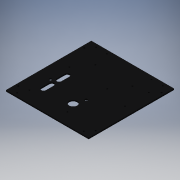
# Autodesk Inventor part: SwarmieTopPlate
Saved by Autodesk Inventor 2016 (Build 200138000, 138)
## iProperties
Created: 2015-05-25
Part Number: SwarmieTopPlate
Material: Generic
Document SubType Name: Modeling
Designer: Karl
Density: 1 g/cm^3
Appearance: Glossy - Black
Author: Karl
Autodesk Inventor part; units mm, degrees
ref_plane "YZ Plane" through (0, 0, 0) normal (1, 0, 0) x (0, 1, 0)
ref_plane "XZ Plane" through (0, 0, 0) normal (0, 1, 0) x (-1, 0, 0)
ref_plane "XY Plane" through (0, 0, 0) normal (0, 0, 1) x (1, 0, 0)
sketch "Sketch1" plane through (0, 0, 0) normal (0, 1, 0) x (-1, 0, 0)
  line L0 (98.0186, -101.2063) -> (-98.0186, -101.2063)
  line L1 (-98.0186, -101.2063) -> (-98.0186, 101.2063)
  line L2 (-98.0186, 101.2063) -> (98.0186, 101.2063)
  line L3 (98.0186, 101.2063) -> (98.0186, -101.2063)
  line L4 (98.0186, -101.2063) -> (-98.0186, 101.2063) construction
  line L5 (-98.0186, -101.2063) -> (98.0186, 101.2063) construction
  point P0 (0, 0)
  dimension "d0" = 196.0372
  dimension "d1" = 202.4126
  constraints: 12 end point, 2 midpoint, 2 parallel, 1 horizontal, 1 perpendicular
  measures "d0" distance of L1.end L2.end
  measures "d1" distance of L0.end L1.end
extrude "Extrusion1" add sketch "Sketch1" along normal blind 3
sketch "Sketch2" plane through (0, 3, 0) normal (0, 1, 0) x (1, 0, 0)
  line L0 (98.0186, 101.2063) -> (-98.0186, 101.2063) projected
  line L1 (-98.0186, 101.2063) -> (-98.0186, -101.2063) projected
  line L2 (-98.0186, -101.2063) -> (98.0186, -101.2063) projected
  line L3 (98.0186, -101.2063) -> (98.0186, 101.2063) projected
  point P0 (0, 0)
  point P1 (-91.6686, 78.0923)
  point P2 (91.6686, 78.0923)
  point P3 (-91.6686, -78.0923)
  point P4 (91.6686, -78.0923)
  dimension "d4" = 23.114
  dimension "d5" = 23.114
  dimension "d6" = 6.35
  dimension "d7" = 6.35
  constraints: 2 horizontal alignment, 2 vertical alignment
  measures "d4" distance from line of L0 point (-91.669, 78.092)
  measures "d5" distance from line of L2 point (-91.669, -78.092)
  measures "d6" distance from line of L1 point (-91.669, 78.092)
  measures "d7" distance from line of L3 point (91.669, 78.092)
hole "Hole1" at (-91.6686, 3, -78.0923) at (91.6686, 3, -78.0923) at (-91.6686, 3, 78.0923) at (91.6686, 3, 78.0923) direction (0, -1, 0) diameter 3.81 end through all
sketch "Sketch5" plane through (0, 3, 0) normal (0, 1, 0) x (1, 0, 0)
  line L0 (-98.0186, 101.2063) -> (-98.0186, -101.2063) projected
  line L1 (-98.0186, -101.2063) -> (98.0186, -101.2063) projected
  point P0 (0, 0)
  point P1 (-70.0786, -73.2663)
  point P2 (19.8374, -73.2663)
  point P3 (19.8374, 21.2217)
  point P4 (-70.0786, 21.2217)
  dimension "d44" = 27.94
  dimension "d45" = 27.94
  dimension "d46" = 89.916
  dimension "d47" = 94.488
  constraints: 2 horizontal alignment, 2 vertical alignment
  measures "d44" distance from line of L1 point (-70.079, -73.266)
  measures "d45" distance from line of L0 point (-70.079, -73.266)
  measures "d46" distance of point (19.837, -73.266) point (-70.079, -73.266)
  measures "d47" distance of point (-70.079, 21.222) point (-70.079, -73.266)
hole "Hole4" at (-70.0786, 3, 73.2663) at (19.8374, 3, 73.2663) at (19.8374, 3, -21.2217) at (-70.0786, 3, -21.2217) direction (0, -1, 0) diameter 3.302 end through all
sketch "Sketch6" plane through (0, 3, 0) normal (0, 1, 0) x (1, 0, 0)
  circle A0 centre (-70.0786, -73.2663) radius 1.651 projected
  circle A1 centre (19.8374, -73.2663) radius 1.651 projected
  point P0 (0, 0)
  point P1 (-67.2846, -26.0223)
  point P2 (17.0434, -26.0223)
  dimension "d55" = 2.794
  dimension "d56" = 2.794
  dimension "d57" = 47.244
  constraints: 1 horizontal alignment
  measures "d55" horizontal distance of point (-67.285, -26.022) A0.centre
  measures "d56" horizontal distance of A1.centre point (17.043, -26.022)
  measures "d57" vertical distance of point (-67.285, -26.022) A0.centre
hole "Hole5" at (-67.2846, 3, 26.0223) at (17.0434, 3, 26.0223) direction (0, -1, 0) diameter 6.35 end through all
sketch "Sketch10" plane through (0, 3, 0) normal (0, 1, 0) x (1, 0, 0)
  line L0 (98.0186, 101.2063) -> (-98.0186, 101.2063) projected
  line L1 (98.0186, -101.2063) -> (98.0186, 101.2063) projected
  line L2 (0, 56.7563) -> (0, 92.8243)
  point P0 (0, 0)
  point P1 (-52.8574, 92.8243)
  point P2 (-43.9674, 56.7563)
  point P3 (52.8574, 92.8243)
  point P4 (43.9674, 56.7563)
  dimension "d91" = 52.8574
  dimension "d92" = 8.382
  dimension "d93" = 36.068
  dimension "d94" = 8.89
  constraints: 2 end point, 2 symmetric about line, 1 parallel
  measures "d91" horizontal distance of point (-52.857, 92.824) point (0, 0)
  measures "d92" distance from line of L0 point (-52.857, 92.824)
  measures "d93" vertical distance of point (-43.967, 56.756) point (-52.857, 92.824)
  measures "d94" horizontal distance of point (-43.967, 56.756) point (-52.857, 92.824)
hole "Hole8" at (-52.8574, 3, -92.8243) at (-43.9674, 3, -56.7563) at (52.8574, 3, -92.8243) at (43.9674, 3, -56.7563) direction (0, -1, 0) diameter 3.302 end through all
sketch "Sketch11" plane through (0, 3, 0) normal (0, 1, 0) x (1, 0, 0)
  line L0 (98.0186, 101.2063) -> (-98.0186, 101.2063) projected
  line L1 (98.0186, -101.2063) -> (98.0186, 101.2063) projected
  point P0 (0, 0)
  point P1 (76.4286, 6.5913)
  point P2 (76.4286, 63.1063)
  dimension "d103" = 56.515
  dimension "d111" = 38.1
  dimension "d123" = 21.59
  constraints: 1 vertical alignment
  measures "d103" distance of point (76.429, 6.591) point (76.429, 63.106)
  measures "d111" distance from line of L0 point (76.429, 63.106)
  measures "d123" distance from line of L1 point (76.429, 6.591)
hole "Hole9" at (76.4286, 3, -6.5913) at (76.4286, 3, -63.1063) direction (0, -1, 0) diameter 3.302 end through all
sketch "Sketch12" plane through (0, 3, 0) normal (0, 1, 0) x (1, 0, 0)
  line L0 (98.0186, 101.2063) -> (-98.0186, 101.2063) projected
  line L1 (-98.0186, 101.2063) -> (-98.0186, -101.2063) projected
  line L2 (-98.0186, -101.2063) -> (98.0186, -101.2063) projected
  line L3 (98.0186, -101.2063) -> (98.0186, 101.2063) projected
  point P0 (0, 0)
  point P1 (-78.9686, -93.5863)
  point P2 (78.9686, -93.5863)
  point P3 (78.9686, 93.5863)
  point P4 (-78.9686, 93.5863)
  dimension "d112" = 7.62
  dimension "d113" = 19.05
  dimension "d114" = 7.62
  dimension "d115" = 19.05
  constraints: 2 horizontal alignment, 2 vertical alignment
  measures "d112" distance from line of L2 point (-78.969, -93.586)
  measures "d113" distance from line of L1 point (-78.969, -93.586)
  measures "d114" distance from line of L0 point (-78.969, 93.586)
  measures "d115" distance from line of L3 point (78.969, 93.586)
hole "Hole10" at (-78.9686, 3, 93.5863) at (78.9686, 3, 93.5863) at (78.9686, 3, -93.5863) at (-78.9686, 3, -93.5863) direction (0, -1, 0) diameter 3.302 end through all
sketch "Sketch13" plane through (0, 3, 0) normal (0, 1, 0) x (1, 0, 0)
  line L0 (-55.88, 2.1463) -> (-55.88, -17.2847) construction
  line L1 (-61.4426, 2.1463) -> (-61.4426, -17.2847)
  line L2 (-50.3174, -17.2847) -> (-50.3174, 2.1463)
  arc A0 (-50.3174, 2.1463) -> (-61.4426, 2.1463) centre (-55.88, 2.1463) ccw
  arc A1 (-61.4426, -17.2847) -> (-50.3174, -17.2847) centre (-55.88, -17.2847) ccw
  circle A2 centre (-70.0786, 21.2217) radius 1.651 projected
  line L3 (-55.88, -34.7599) -> (-55.88, -54.1909) construction
  line L4 (-61.4426, -34.7599) -> (-61.4426, -54.1909)
  line L5 (-50.3174, -54.1909) -> (-50.3174, -34.7599)
  arc A3 (-50.3174, -34.7599) -> (-61.4426, -34.7599) centre (-55.88, -34.7599) ccw
  arc A4 (-61.4426, -54.1909) -> (-50.3174, -54.1909) centre (-55.88, -54.1909) ccw
  point P0 (0, 0)
  point P1 (-55.88, -7.5692)
  point P2 (-55.88, -44.4754)
  dimension "d124" = 14.1986
  dimension "d125" = 11.1252
  dimension "d126" = 19.0754
  dimension "d127" = 19.431
  dimension "d128" = 19.431
  dimension "d129" = 11.1252
  dimension "d138" = 17.4752
  constraints: 16 end point, 8 point on circle, 8 tangent, 4 centre point, 2 midpoint, 2 parallel, 2 vertical, 1 collinear
  measures "d124" horizontal distance of A2.centre L0.start
  measures "d125" distance between parallel lines of L1 L2
  measures "d126" vertical distance of A2.centre L0.start
  measures "d127" distance of L2.start L2.end
  measures "d128" distance of L5.start L5.end
  measures "d129" distance between parallel lines of L5 L4
  measures "d138" distance of L3.start L0.end
extrude "Extrusion3" cut sketch "Sketch13" against normal through all contours A0 L2 A1 L1 | A3 L5 A4 L4
sketch "Sketch14" plane through (0, 3, 0) normal (0, 1, 0) x (1, 0, 0)
  circle A0 centre (8.6614, -48.4759) radius 9.652
  circle A1 centre (19.8374, -73.2663) radius 1.651 projected
  point P0 (0, 0)
  dimension "d133" = 19.304
  dimension "d134" = 11.176
  dimension "d135" = 24.7904
  constraints: 1 centre point
  measures "d133" diameter of A0
  measures "d134" horizontal distance of A1.centre A0.centre
  measures "d135" vertical distance of A1.centre A0.centre
extrude "Extrusion4" cut sketch "Sketch14" against normal through all contours A0
equation "\"d128\" = d127"
equation "\"d129\" = d125"
body "Solid1"
